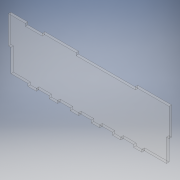
# Autodesk Inventor part: back
Saved by Autodesk Inventor 2017.2 (Build 212233000, 233)
## iProperties
Created: 2017-06-02
Part Number: back
Material: Generic
Document SubType Name: Modeling
Designer: SandeepSH
Density: 1 g/cm^3
Appearance: Polycarbonate - Clear
Author: SandeepSH
Autodesk Inventor part; units mm, degrees
ref_plane "YZ Plane" through (0, 0, 0) normal (1, 0, 0) x (0, 1, 0)
ref_plane "XZ Plane" through (0, 0, 0) normal (0, 1, 0) x (-1, 0, 0)
ref_plane "XY Plane" through (0, 0, 0) normal (0, 0, 1) x (1, 0, 0)
sketch "Sketch1" plane through (0, 0, 0) normal (0, 0, 1) x (1, 0, 0)
  line L0 (-95, -31.5) -> (95, -31.5)
  line L1 (95, -31.5) -> (95, 31.5)
  line L2 (95, 31.5) -> (-95, 31.5)
  line L3 (-95, 31.5) -> (-95, -31.5)
  line L4 (-95, -31.5) -> (95, 31.5) construction
  line L5 (95, -31.5) -> (-95, 31.5) construction
  point P0 (0, 0)
  dimension "d0" = 190
  dimension "d1" = 63
  constraints: 12 end point, 2 midpoint, 2 parallel, 1 horizontal, 1 perpendicular
  measures "d0" distance of L2.end L1.end
  measures "d1" distance of L1.end L0.end
extrude "Extrusion1" add sketch "Sketch1" along normal blind 3
sketch "Sketch2" plane through (0, 0, 3) normal (0, 0, 1) x (1, 0, 0)
  line L0 (-95, 31.5) -> (-95, -31.5) projected
  line L1 (-95, -31.5) -> (-92, -31.5)
  line L2 (-92, -31.5) -> (-92, -1.5)
  line L3 (-92, -1.5) -> (-95, -1.5)
  line L4 (-95, -1.5) -> (-95, -31.5)
  line L5 (-92, -31.5) -> (-72, -31.5)
  line L6 (-72, -31.5) -> (-72, -28.5)
  line L7 (-72, -28.5) -> (-92, -28.5)
  line L8 (-92, -28.5) -> (-92, -31.5)
  line L9 (-95, -31.5) -> (95, -31.5) projected
  line L10 (-62, -31.5) -> (-47, -31.5)
  line L11 (-47, -31.5) -> (-47, -28.5)
  line L12 (-47, -28.5) -> (-62, -28.5)
  line L13 (-62, -28.5) -> (-62, -31.5)
  line L14 (-37, -31.5) -> (-22, -31.5)
  line L15 (-22, -31.5) -> (-22, -28.5)
  line L16 (-22, -28.5) -> (-37, -28.5)
  line L17 (-37, -28.5) -> (-37, -31.5)
  line L18 (-12, -31.5) -> (3, -31.5)
  line L19 (3, -31.5) -> (3, -28.5)
  line L20 (3, -28.5) -> (-12, -28.5)
  line L21 (-12, -28.5) -> (-12, -31.5)
  line L22 (13, -31.5) -> (28, -31.5)
  line L23 (28, -31.5) -> (28, -28.5)
  line L24 (28, -28.5) -> (13, -28.5)
  line L25 (13, -28.5) -> (13, -31.5)
  line L26 (38, -31.5) -> (53, -31.5)
  line L27 (53, -31.5) -> (53, -28.5)
  line L28 (53, -28.5) -> (38, -28.5)
  line L29 (38, -28.5) -> (38, -31.5)
  line L30 (95, -31.5) -> (92, -31.5)
  line L31 (92, -31.5) -> (92, -1.5)
  line L32 (92, -1.5) -> (95, -1.5)
  line L33 (95, -1.5) -> (95, -31.5)
  line L34 (92, -31.5) -> (63, -31.5)
  line L35 (63, -31.5) -> (63, -28.5)
  line L36 (63, -28.5) -> (92, -28.5)
  line L37 (92, -28.5) -> (92, -31.5)
  point P0 (0, 0)
  dimension "d4" = 3
  dimension "d5" = 30
  dimension "d7" = 20
  dimension "d8" = 3
  dimension "d9" = 15
  dimension "d10" = 15
  dimension "d11" = 15
  dimension "d12" = 15
  dimension "d13" = 15
  dimension "d14" = 10
  dimension "d15" = 10
  dimension "d16" = 10
  dimension "d17" = 10
  dimension "d18" = 10
  dimension "d20" = 3
  dimension "d21" = 30
  dimension "d22" = 10
  constraints: 72 end point, 18 parallel, 10 point on line, 9 horizontal, 9 perpendicular
  measures "d4" distance of L3.end L2.end
  measures "d5" distance of L2.end L1.end
  measures "d7" distance of L7.end L6.end
  measures "d8" distance of L6.end L5.end
  measures "d9" distance of L12.end L11.end
  measures "d10" distance of L16.end L15.end
  measures "d11" distance of L20.end L19.end
  measures "d12" distance of L24.end L23.end
  measures "d13" distance of L28.end L27.end
  measures "d14" distance between parallel lines of L29 L23
  measures "d15" distance from line of L22.start L19
  measures "d16" distance between parallel lines of L21 L15
  measures "d17" distance between parallel lines of L17 L11
  measures "d18" distance between parallel lines of L13 L6
  measures "d20" distance of L31.end L32.end
  measures "d21" distance of L30.end L31.end
  measures "d22" distance between parallel lines of L35 L27
extrude "Extrusion2" cut sketch "Sketch2" against normal through all
sketch "Sketch3" plane through (0, 0, 3) normal (0, 0, 1) x (1, 0, 0)
  line L0 (95, 31.5) -> (-95, 31.5) projected
  line L1 (-15, 31.5) -> (55, 31.5)
  line L2 (55, 31.5) -> (55, 28.5)
  line L3 (55, 28.5) -> (-15, 28.5)
  line L4 (-15, 28.5) -> (-15, 31.5)
  line L5 (95, -1.5) -> (95, 31.5) projected
  line L6 (-75, 31.5) -> (-55, 31.5)
  line L7 (-55, 31.5) -> (-55, 28.5)
  line L8 (-55, 28.5) -> (-75, 28.5)
  line L9 (-75, 28.5) -> (-75, 31.5)
  line L10 (-95, 31.5) -> (-95, -1.5) projected
  point P0 (0, 0)
  dimension "d25" = 3
  dimension "d26" = 40
  dimension "d27" = 70
  dimension "d28" = 20
  dimension "d29" = 20
  constraints: 16 end point, 4 parallel, 2 horizontal, 2 perpendicular, 2 point on line
  measures "d25" distance of L1.end L2.end
  measures "d26" distance between parallel lines of L5 L2
  measures "d27" distance between parallel lines of L2 L4
  measures "d28" distance of L7.end L8.end
  measures "d29" distance between parallel lines of L9 L10
extrude "Extrusion3" cut sketch "Sketch3" against normal through all
equation "\"d10\" = d9"
equation "\"d11\" = d10"
equation "\"d12\" = d11"
equation "\"d13\" = d12"
equation "\"d15\" = d14"
equation "\"d16\" = d15"
equation "\"d17\" = d16"
equation "\"d18\" = d16"
equation "\"d22\" = d14"
body "Solid1"
